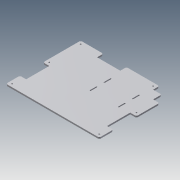
# Autodesk Inventor part: ProjectorPlateFront
Saved by Autodesk Inventor 2014 (Build 180170000, 170)
## iProperties
Created: 2014-08-10
Part Number: ProjectorPlateFront
Material: Generic
Document SubType Name: Modeling
Designer: Peele
Density: 1 g/cm^3
Appearance: White
Author: Peele
Autodesk Inventor part; units mm, degrees
ref_plane "YZ Plane" through (0, 0, 0) normal (1, 0, 0) x (0, 1, 0)
ref_plane "XZ Plane" through (0, 0, 0) normal (0, 1, 0) x (-1, 0, 0)
ref_plane "XY Plane" through (0, 0, 0) normal (0, 0, 1) x (1, 0, 0)
sketch "Sketch1" plane through (0, 0, 0) normal (0, 0, 1) x (1, 0, 0)
  line L0 (-187.5, -150) -> (187.5, -150)
  line L1 (187.5, -150) -> (187.5, 150)
  line L2 (187.5, 150) -> (-187.5, 150)
  line L3 (-187.5, 150) -> (-187.5, -150)
  line L4 (-187.5, -150) -> (187.5, 150) construction
  line L5 (187.5, -150) -> (-187.5, 150) construction
  point P0 (0, 0)
  dimension "d0" = 375
  dimension "d1" = 300
  constraints: 12 end point, 2 midpoint, 2 parallel, 1 horizontal, 1 perpendicular
  measures "d0" distance of L0.start L0.end
  measures "d1" distance of L0.end L1.end
extrude "Extrusion1" add sketch "Sketch1" along normal blind 6
sketch "Sketch6" plane through (0, 0, 0) normal (0, 0, -1) x (-1, 0, 0)
  line L0 (-187.5, 150) -> (-162.5, 150)
  line L1 (-162.5, 150) -> (-162.5, 125)
  line L2 (-162.5, 125) -> (-187.5, 125)
  line L3 (-187.5, 125) -> (-187.5, 150)
  line L4 (187.5, 150) -> (187.5, -150) projected
  line L5 (-187.5, 150) -> (187.5, 150) projected
  line L6 (-187.5, -150) -> (-187.5, 150) projected
  line L7 (-187.5, -35) -> (-162.5, -35)
  line L8 (-162.5, -35) -> (-162.5, -60)
  line L9 (-162.5, -60) -> (-187.5, -60)
  line L10 (-187.5, -60) -> (-187.5, -35)
  line L11 (187.5, -35) -> (162.5, -35)
  line L12 (162.5, -35) -> (162.5, -60)
  line L13 (162.5, -60) -> (187.5, -60)
  line L14 (187.5, -60) -> (187.5, -35)
  line L15 (62.5, 150) -> (37.5, 150)
  line L16 (37.5, 150) -> (37.5, 125)
  line L17 (37.5, 125) -> (62.5, 125)
  line L18 (62.5, 125) -> (62.5, 150)
  point P0 (0, 0)
  dimension "d22" = 25
  dimension "d25" = 160
  dimension "d26" = 200
  constraints: 32 end point, 8 parallel, 7 equal length, 4 horizontal, 4 perpendicular, 3 point on line, 1 collinear
  measures "d22" distance of L0.start L0.end
  measures "d25" distance between parallel lines of L2 L7
  measures "d26" distance between parallel lines of L1 L16
extrude "Extrusion6" cut sketch "Sketch6" against normal through all
sketch "Sketch7" plane through (0, 0, 0) normal (0, 0, -1) x (-1, 0, 0)
  line L0 (-162.5, -60) -> (-187.5, -60) projected
  line L1 (-187.5, -150) -> (-187.5, -60) projected
  line L2 (187.5, -60) -> (187.5, -150) projected
  line L3 (187.5, -60) -> (162.5, -60) projected
  line L4 (62.5, 150) -> (187.5, 150) projected
  line L5 (37.5, 125) -> (37.5, 150) projected
  line L6 (-162.5, 150) -> (37.5, 150) projected
  line L7 (-162.5, 125) -> (-187.5, 125) projected
  line L8 (-187.5, -35) -> (-187.5, 125) projected
  line L9 (-162.5, 125) -> (-187.5, 125)
  line L10 (-187.5, 125) -> (-187.5, 91)
  line L11 (-187.5, 91) -> (-162.5, 91)
  line L12 (-162.5, 91) -> (-162.5, 125)
  line L13 (-162.5, 125) -> (-128.5, 125)
  line L14 (-128.5, 125) -> (-128.5, 150)
  line L15 (-128.5, 150) -> (-162.5, 150)
  line L16 (-162.5, 150) -> (-162.5, 125)
  line L17 (37.5, 125) -> (3.5, 125)
  line L18 (3.5, 125) -> (3.5, 150)
  line L19 (3.5, 150) -> (37.5, 150)
  line L20 (37.5, 150) -> (37.5, 125)
  line L21 (62.5, 125) -> (96.5, 125)
  line L22 (96.5, 125) -> (96.5, 150)
  line L23 (96.5, 150) -> (62.5, 150)
  line L24 (62.5, 150) -> (62.5, 125)
  line L25 (187.5, -35) -> (162.5, -35)
  line L26 (162.5, -35) -> (162.5, -1)
  line L27 (162.5, -1) -> (187.5, -1)
  line L28 (187.5, -1) -> (187.5, -35)
  line L29 (162.5, -60) -> (187.5, -60)
  line L30 (187.5, -60) -> (187.5, -94)
  line L31 (187.5, -94) -> (162.5, -94)
  line L32 (162.5, -94) -> (162.5, -60)
  line L33 (-162.5, -60) -> (-187.5, -60)
  line L34 (-187.5, -60) -> (-187.5, -94)
  line L35 (-187.5, -94) -> (-162.5, -94)
  line L36 (-162.5, -94) -> (-162.5, -60)
  line L37 (-162.5, -35) -> (-187.5, -35)
  line L38 (-187.5, -35) -> (-187.5, -1)
  line L39 (-187.5, -1) -> (-162.5, -1)
  line L40 (-162.5, -1) -> (-162.5, -35)
  point P0 (0, 0)
  dimension "d31" = 34
  constraints: 64 end point, 16 parallel, 8 equal length, 8 horizontal, 8 perpendicular, 7 point on line
  measures "d31" distance of L7.start L13.end
extrude "Extrusion7" cut sketch "Sketch7" against normal through all
sketch "Sketch8" plane through (0, 0, 6) normal (0, 0, 1) x (1, 0, 0)
  line L0 (187.5, -150) -> (187.5, 150) projected
  line L1 (128.5, 125) -> (128.5, 150) projected
  line L2 (187.5, 150) -> (-187.5, 150) projected
  line L3 (-187.5, -1) -> (-162.5, -1) projected
  line L4 (-162.5, -94) -> (-187.5, -94) projected
  line L5 (-187.5, -150) -> (187.5, -150) projected
  circle A0 centre (-175, 137.5) radius 2.7
  circle A1 centre (-175, 11.5) radius 2.7
  circle A2 centre (-175, -137.5) radius 2.7
  circle A3 centre (175, -137.5) radius 2.7
  circle A4 centre (175, 11.5) radius 2.7
  circle A5 centre (116, 137.5) radius 2.7
  line L6 (-175, -137.5) -> (-175, -94) construction
  point P0 (187.5, -1)
  point P1 (187.5, 91)
  point P2 (-96.5, 150)
  point P3 (0, 0)
  dimension "d32" = 12.5
  dimension "d33" = 12.5
  dimension "d34" = 12.5
  dimension "d35" = 12.5
  dimension "d36" = 12.5
  dimension "d37" = 5.4
  constraints: 6 centre point, 5 equal radius, 3 horizontal alignment, 3 vertical alignment, 2 end point, 1 midpoint, 1 vertical
  measures "d32" distance from line of A1.centre L3
  measures "d33" distance from line of A0.centre L2
  measures "d34" distance from line of A5.centre L1
  measures "d35" distance from line of A4.centre L0
  measures "d36" distance from line of A3.centre L5
  measures "d37" diameter of A0
extrude "Extrusion8" cut sketch "Sketch8" against normal blind 10
sketch "Sketch9" plane through (0, 0, 6) normal (0, 0, 1) x (1, 0, 0)
  line L0 (187.5, -150) -> (187.5, 150) projected
  line L1 (187.5, 150) -> (-187.5, 150) projected
  line L2 (-3.5, 125) -> (-96.5, 125) projected
  line L3 (187.5, -94) -> (162.5, -94) projected
  line L4 (5.5, 77.5) -> (5.5, 52.5) construction
  line L5 (3.35, 77.5) -> (3.35, 52.5)
  line L6 (7.65, 52.5) -> (7.65, 77.5)
  arc A0 (7.65, 77.5) -> (3.35, 77.5) centre (5.5, 77.5) ccw
  arc A1 (3.35, 52.5) -> (7.65, 52.5) centre (5.5, 52.5) ccw
  line L7 (5.5, -4.1) -> (5.5, 20.9) construction
  line L8 (3.35, -4.1) -> (3.35, 20.9)
  line L9 (7.65, 20.9) -> (7.65, -4.1)
  arc A2 (3.35, -4.1) -> (7.65, -4.1) centre (5.5, -4.1) ccw
  arc A3 (7.65, 20.9) -> (3.35, 20.9) centre (5.5, 20.9) ccw
  line L10 (119.5, 77.5) -> (119.5, 52.5) construction
  line L11 (117.35, 77.5) -> (117.35, 52.5)
  line L12 (121.65, 52.5) -> (121.65, 77.5)
  arc A4 (121.65, 77.5) -> (117.35, 77.5) centre (119.5, 77.5) ccw
  arc A5 (117.35, 52.5) -> (121.65, 52.5) centre (119.5, 52.5) ccw
  line L13 (119.5, 20.9) -> (119.5, -4.1) construction
  line L14 (117.35, 20.9) -> (117.35, -4.1)
  line L15 (121.65, -4.1) -> (121.65, 20.9)
  arc A6 (121.65, 20.9) -> (117.35, 20.9) centre (119.5, 20.9) ccw
  arc A7 (117.35, -4.1) -> (121.65, -4.1) centre (119.5, -4.1) ccw
  line L16 (-50, 125) -> (-50, -47.5) construction
  line L17 (-50, -47.5) -> (175, -47.5) construction
  line L18 (175, -47.5) -> (175, -94) construction
  line L19 (5.5, 8.4) -> (119.5, 8.4) construction
  line L20 (62.5, 8.4) -> (62.5, -47.5) construction
  point P0 (187.5, -1)
  point P1 (187.5, 91)
  point P2 (128.5, 150)
  point P3 (-3.5, 150)
  point P4 (0, 0)
  point P5 (5.5, 65)
  point P6 (119.5, 65)
  point P7 (-37.5, 125)
  point P8 (-62.5, 125)
  dimension "d40" = 114
  dimension "d41" = 2.15
  dimension "d42" = 56.6
  dimension "d43" = 25
  dimension "d44" = 85
  constraints: 42 end point, 16 point on circle, 16 tangent, 9 parallel, 8 centre point, 8 midpoint, 3 equal length, 3 equal radius, 2 collinear, 2 horizontal alignment, 2 vertical, 1 horizontal, 1 perpendicular
  measures "d40" distance between parallel lines of L4 L10
  measures "d41" radius of A4
  measures "d42" distance of point (119.5, 65) L19.end
  measures "d43" distance of L15.start L15.end
  measures "d44" distance from line of L1 point (119.5, 65)
extrude "Extrusion9" cut sketch "Sketch9" against normal blind 10
fillet "Fillet3" radius 6 12 edges at (187.5, -150, 3) (187.5, -94, 3) (187.5, -1, 3) (187.5, 91, 3) (162.5, 125, 3) (128.5, 150, 3) (-3.5, 150, 3) (-96.5, 150, 3) (-187.5, 150, 3) (-187.5, -94, 3) (-187.5, -150, 3) (-187.5, -1, 3)
equation "\"d33\" = d32"
equation "\"d34\" = d32"
equation "\"d35\" = d33"
equation "\"d36\" = d32"
body "Solid1"
